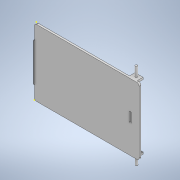
# Autodesk Inventor part: base
Saved by Autodesk Inventor 2022 (Build 260153000, 153)
## iProperties
Created: 2022-08-22
Part Number: base
Material: Generic
Document SubType Name: Modeling
Designer: Sachin
Density: 1 g/cm^3
Appearance: Default
Author: Sachin
Autodesk Inventor part; units mm, degrees
ref_plane "YZ Plane" through (0, 0, 0) normal (1, 0, 0) x (0, 1, 0)
ref_plane "XZ Plane" through (0, 0, 0) normal (0, 1, 0) x (-1, 0, 0)
ref_plane "XY Plane" through (0, 0, 0) normal (0, 0, 1) x (1, 0, 0)
sketch "Sketch1" plane through (0, 0, 0) normal (0, 0, 1) x (1, 0, 0)
  point P0 (0, 0)
sketch "Sketch2" plane through (0, 0, 0) normal (0, 0, 1) x (1, 0, 0)
  line L0 (0, 0) -> (279.4, 0)
  line L1 (279.4, 0) -> (279.4, 177.8)
  line L2 (279.4, 177.8) -> (0, 177.8)
  line L3 (0, 177.8) -> (0, 0)
  constraints: 8 end point, 2 parallel, 1 horizontal, 1 perpendicular
extrude "Extrusion1" add sketch "Sketch2" along normal blind 5
fillet "Fillet1" radius 6 4 edges at (0, 177.8, 2.5) (0, 0, 2.5) (279.4, 0, 2.5) (279.4, 177.8, 2.5)
sketch "Sketch3" plane through (0, 0, 5) normal (0, 0, 1) x (1, 0, 0)
  line L0 (258.2444, 76.2) -> (253.2444, 76.2)
  line L1 (253.2444, 76.2) -> (253.2444, 101.6)
  line L2 (253.2444, 101.6) -> (258.2444, 101.6)
  line L3 (258.2444, 101.6) -> (258.2444, 76.2)
  line L4 (6, 0) -> (273.4, 0) projected
  point P0 (0, 0)
  dimension "d5" = 5
  dimension "d6" = 25.4
  dimension "d7" = 76.2
  constraints: 8 end point, 2 parallel, 1 horizontal, 1 perpendicular
  measures "d5" distance of L1.end L2.end
  measures "d6" distance of L2.end L0.start
  measures "d7" distance between parallel lines of L4 L0
extrude "Extrusion2" cut sketch "Sketch3" against normal blind 2
sketch "Sketch4" plane through (0, 0, 5) normal (0, 0, 1) x (1, 0, 0)
  point P0 (0, 0)
sketch "Sketch5" plane through (0, 0, 0) normal (0, 0, -1) x (-1, 0, 0)
  line L0 (-273.4, 177.8) -> (-6, 177.8) projected
  line L1 (-270.0239, 177.8) -> (-248.6645, 177.8)
  line L2 (-248.6645, 177.8) -> (-248.6645, 172.369)
  line L3 (-248.6645, 172.369) -> (-270.0239, 172.369)
  line L4 (-270.0239, 172.369) -> (-270.0239, 177.8)
  line L5 (-6, 0) -> (-273.4, 0) projected
  line L6 (-270.0239, 0) -> (-248.6645, 0)
  line L7 (-248.6645, 0) -> (-248.6645, 5.4307)
  line L8 (-248.6645, 5.4307) -> (-270.0239, 5.4307)
  line L9 (-270.0239, 5.4307) -> (-270.0239, 0)
  point P0 (0, 0)
  dimension "d10" = 5.4307
  dimension "d11" = 5.431
  constraints: 16 end point, 4 parallel, 4 point on line, 2 horizontal, 2 perpendicular
  measures "d10" distance between parallel lines of L5 L8
  measures "d11" distance between parallel lines of L3 L0
extrude "Extrusion3" add sketch "Sketch5" along normal blind 15
sketch "Sketch6" plane through (6, 177.8, 5) normal (0, 1, 0) x (1, 0, 0)
  point P0 (-6, 5)
sketch "Sketch7" plane through (6, 177.8, 5) normal (0, 1, 0) x (1, 0, 0)
  circle A0 centre (253.4743, 12.5024) radius 3
  point P0 (-6, 5)
  dimension "d14" = 6
  constraints: 1 centre point
  measures "d14" diameter of A0
sketch "Sketch8" plane through (6, 0, 5) normal (0, -1, 0) x (1, 0, 0)
  circle A0 centre (254.3422, -12.325) radius 3
  point P0 (-6, -5)
  dimension "d15" = 6
  constraints: 1 centre point
  measures "d15" diameter of A0
extrude "Extrusion4" add sketch "Sketch8" along normal blind 25.4
extrude "Extrusion5" add sketch "Sketch7" along normal blind 25.4
sketch "Sketch9" plane through (0, 0, 5) normal (0, 0, 1) x (1, 0, 0)
  line L0 (0, 171.8) -> (0, 6) projected
  line L1 (0, 139.7) -> (1.4974, 139.7)
  line L2 (1.4974, 139.7) -> (1.4974, 38.1)
  line L3 (1.4974, 38.1) -> (0, 38.1)
  line L4 (0, 38.1) -> (0, 139.7)
  line L5 (6, 0) -> (273.4, 0) projected
  line L6 (273.4, 177.8) -> (6, 177.8) projected
  point P0 (0, 0)
  point P1 (0, 38.1)
  dimension "d20" = 38.1
  dimension "d21" = 38.1
  constraints: 8 end point, 2 parallel, 1 horizontal, 1 perpendicular, 1 point on line
  measures "d20" distance between parallel lines of L5 L3
  measures "d21" distance between parallel lines of L1 L6
extrude "Extrusion6" add sketch "Sketch9" along normal blind 2.5
sketch "Sketch13" plane through (0, 0, 0) normal (0, 0, -1) x (-1, 0, 0)
  circle A0 centre (-25.8349, 40.8578) radius 1
  point P0 (0, 0)
  dimension "d32" = 2
  constraints: 1 centre point
  measures "d32" diameter of A0
extrude "Extrusion8" add sketch "Sketch13" along normal blind 5
sketch "Sketch14" plane through (0, 0, 0) normal (0, 0, -1) x (-1, 0, 0)
  circle A0 centre (-24.7974, 137) radius 1
  line L0 (-248.6645, 177.8) -> (-6, 177.8) projected
  line L1 (-1.4974, 139.7) -> (-1.4974, 38.1) projected
  point P0 (0, 0)
  dimension "d35" = 2
  dimension "d36" = 40.8
  dimension "d37" = 23.3
  constraints: 1 centre point
  measures "d35" diameter of A0
  measures "d36" distance from line of A0.centre L0
  measures "d37" distance from line of A0.centre L1
extrude "Extrusion9" add sketch "Sketch14" along normal blind 5
sketch "Sketch15" plane through (0, 0, 0) normal (0, 0, -1) x (-1, 0, 0)
  point P0 (0, 0)
sketch "Sketch16" plane through (0, 0, 5) normal (0, 0, 1) x (1, 0, 0)
  point P0 (0, 0)
body "Solid1"
